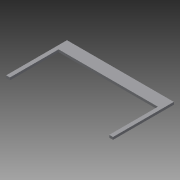
# Autodesk Inventor part: Fork2DimTest
Saved by Autodesk Inventor 2014 SP1 (Build 180222100, 222)
## iProperties
Created: 2017-01-17
Part Number: Fork2DimTest
Material: Generic
Document SubType Name: Modeling
Designer: danielsikar
Density: 1 g/cm^3
Appearance: Default
Author: danielsikar
Autodesk Inventor part; units mm, degrees
ref_plane "YZ Plane" through (0, 0, 0) normal (1, 0, 0) x (0, 1, 0)
ref_plane "XZ Plane" through (0, 0, 0) normal (0, 1, 0) x (-1, 0, 0)
ref_plane "XY Plane" through (0, 0, 0) normal (0, 0, 1) x (1, 0, 0)
sketch "Sketch1" plane through (0, 0, 0) normal (0, 0, 1) x (1, 0, 0)
  line L0 (-6.8, -3.1) -> (-5.8439, -3.1)
  arc A0 (-5.8439, -5.5) -> (-5.8439, -3.1) centre (-4, -4.3) ccw
  line L1 (-5.8439, -5.5) -> (-6.8, -5.5)
  line L2 (-6.8, -5.5) -> (-6.8, -3.1)
  line L3 (-6.8, -16.9) -> (-6.8, -14.5)
  line L4 (-5.8439, -14.5) -> (-6.8, -14.5)
  arc A1 (-5.8439, -16.9) -> (-5.8439, -14.5) centre (-4, -15.7) ccw
  line L5 (-5.8439, -16.9) -> (-6.8, -16.9)
  arc A2 (47.1, 2) -> (44.1, 5) centre (44.1, 2) ccw
  line L6 (44.1, 5) -> (-5.8, 5)
  arc A3 (-5.8, 5) -> (-8.8, 2) centre (-5.8, 2) ccw
  line L7 (-8.8, -3.3038) -> (-8.8, 2)
  spline S0 degree 3 poles (-11.8, -8.5) (-11.3844, -8.0844) (-10.926, -7.6277) (-10.0868, -6.6554) (-9.7097, -6.1367) (-9.2499, -5.2825) (-9.0837, -4.8972) (-8.8584, -4.0991) (-8.8, -3.6862) (-8.8, -3.3038) knots 0 0 0 0 0.176344 0.176344 0.352688 0.352688 0.467383 0.467383 0.582078 0.582078 0.582078 0.582078
  line L8 (-71, -8.5) -> (-11.8, -8.5)
  arc A4 (-71, -11.5) -> (-71, -8.5) centre (-71.8, -10) ccw
  line L9 (-11.8, -11.5) -> (-71, -11.5)
  spline S1 degree 3 poles (-8.8, -16.6962) (-8.8, -16.3138) (-8.8584, -15.9009) (-9.0837, -15.1028) (-9.2499, -14.7175) (-9.7097, -13.8633) (-10.0868, -13.3446) (-10.926, -12.3723) (-11.3844, -11.9156) (-11.8, -11.5) knots 1.516597 1.516597 1.516597 1.516597 1.631292 1.631292 1.745986 1.745986 1.922331 1.922331 2.098675 2.098675 2.098675 2.098675
  line L10 (-8.8, -17) -> (-8.8, -16.6962)
  arc A5 (-8.8, -17) -> (-5.8, -20) centre (-5.8, -17) ccw
  line L11 (-5.8, -20) -> (0, -20)
  line L12 (0, -20) -> (0, 0)
  line L13 (0, 0) -> (40.3, 0)
  line L14 (40.3, -20) -> (40.3, 0)
  line L15 (47.1, -20) -> (40.3, -20)
  line L16 (47.1, -16.9) -> (47.1, -20)
  line L17 (47.1, -16.9) -> (46.1439, -16.9)
  arc A6 (46.1439, -14.5) -> (46.1439, -16.9) centre (44.3, -15.7) ccw
  line L18 (46.1439, -14.5) -> (47.1, -14.5)
  line L19 (47.1, -5.5) -> (47.1, -14.5)
  line L20 (47.1, -5.5) -> (46.1439, -5.5)
  arc A7 (46.1439, -3.1) -> (46.1439, -5.5) centre (44.3, -4.3) ccw
  line L21 (46.1439, -3.1) -> (47.1, -3.1)
  line L22 (47.1, -3.1) -> (47.1, 2)
  constraints: 46 end point, 16 point on circle, 8 centre point, 4 other
extrude "Extrusion1" add sketch "Sketch1" along normal blind 1
sketch "Sketch2" plane through (0, 0, 1) normal (0, 0, 1) x (1, 0, 0)
  line L0 (-6.8, -14.5) -> (-5.8439, -14.5) projected
  arc A0 (-5.8439, -16.9) -> (-5.8439, -14.5) centre (-4, -15.7) ccw projected
  line L1 (-5.8439, -16.9) -> (-6.8, -16.9) projected
  line L2 (-6.8, -16.9) -> (-6.8, -14.5) projected
  arc A1 (-5.8439, -5.5) -> (-5.8439, -3.1) centre (-4, -4.3) ccw projected
  line L3 (-5.8439, -5.5) -> (-6.8, -5.5) projected
  line L4 (-6.8, -5.5) -> (-6.8, -3.1) projected
  line L5 (-6.8, -3.1) -> (-5.8439, -3.1) projected
  line L6 (-1.8, 10.0452) -> (-75.924, 10.0452)
  line L7 (-75.924, 10.0452) -> (-75.924, -24.7516)
  line L8 (-75.924, -24.7516) -> (-1.8, -24.7516)
  line L9 (-1.8, -24.7516) -> (-1.8, 10.0452)
  line L10 (42.1, 14.1949) -> (61.4451, 14.1949)
  line L11 (61.4451, 14.1949) -> (61.4451, -26.9512)
  line L12 (61.4451, -26.9512) -> (42.1, -26.9512)
  line L13 (42.1, -26.9512) -> (42.1, 14.1949)
  constraints: 16 end point, 4 parallel, 2 horizontal, 2 perpendicular
extrude "Extrusion2" cut sketch "Sketch2" against normal blind 1
sketch "Sketch3" plane through (0, -20, 0) normal (1, 0, 0) x (0, 0, -1)
  line L0 (0, 0) -> (0, 20) projected
  line L1 (0, 20) -> (-1, 20) projected
  line L2 (-1, 0) -> (-1, 20) projected
  line L3 (0, 0) -> (-1, 0) projected
extrude "Extrusion3" cut sketch "Sketch3" against normal blind 0.25
sketch "Sketch4" plane through (40.3, -20, 0) normal (-1, 0, 0) x (0, 0, 1)
  line L0 (0, 20) -> (0, 0) projected
  line L1 (0, 0) -> (1, 0) projected
  line L2 (1, 20) -> (1, 0) projected
  line L3 (0, 20) -> (1, 20) projected
extrude "Extrusion4" cut sketch "Sketch4" against normal blind 0.25
body "Solid1"
